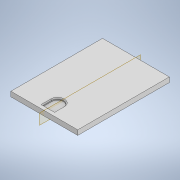
# Autodesk Inventor part: Part2
Saved by Autodesk Inventor 2022.6 (Build 266554010, 554A)
## iProperties
Created: 2025-05-13
Part Number: Part2
Material: Generic
Document SubType Name: Modeling
Designer: khinm
Density: 1 g/cm^3
Appearance: Default
Author: khinm
Autodesk Inventor part; units mm, degrees
ref_plane "XZ Plane" through (0, 0, 0) normal (0, 1, 0) x (-1, 0, 0)
ref_plane "XY Plane" through (0, 0, 0) normal (0, 0, 1) x (1, 0, 0)
sketch "Sketch1" plane through (0, 0, 0) normal (0, 0, 1) x (1, 0, 0)
  line L0 (-37.75, 2.75) -> (37.75, 2.75)
  line L1 (37.75, 2.75) -> (37.75, -2.75)
  line L2 (37.75, -2.75) -> (-37.75, -2.75)
  line L3 (-37.75, -2.75) -> (-37.75, 2.75)
  point P0 (0, 0)
  point P1 (0, 2.75)
  point P2 (-37.75, 0)
  dimension "d0" = 5.5
  dimension "d1" = 75.5
  constraints: 8 end point, 2 midpoint, 2 parallel, 1 horizontal, 1 horizontal alignment, 1 perpendicular, 1 vertical alignment
  measures "d0" distance of L0.end L1.end
  measures "d1" distance of L0.start L0.end
extrude "Extrusion1" add sketch "Sketch1" along normal mid plane 103.5
ref_plane "Work Plane1" through (0, 0, 0) normal (1, 0, 0) x (0, 1, 0)
sketch "Sketch6" plane through (0, 0, 0) normal (1, 0, 0) x (0, 1, 0)
  line L0 (-2.75, 51.75) -> (-2.75, -51.75) projected
  line L1 (-2.75, 49.5) -> (-4.75, 48.3453)
  line L2 (-4.75, 48.3453) -> (-4.75, 47.6547)
  line L3 (-4.75, 47.6547) -> (-2.75, 46.5)
  line L4 (-2.75, 46.5) -> (-2.75, 49.5)
  point P0 (0, 0)
  point P1 (-2.75, 48)
  point P2 (-4.75, 48)
  dimension "d17" = 2.25
  dimension "d18" = 3
  dimension "d19" = 2
  dimension "d20" = 60
  constraints: 8 end point, 2 midpoint, 2 parallel, 1 horizontal alignment, 1 point on line
  measures "d17" distance of L1.start L0.start
  measures "d18" distance of L3.end L1.start
  measures "d19" distance of point (-2.75, 48) point (-4.75, 48)
  measures "d20" angle of L0 L1
extrude "Extrusion4" add sketch "Sketch6" along normal mid plane 59.9
sketch "Sketch7" plane through (-37.75, 2.75, 51.75) normal (0, 1, 0) x (1, 0, 0)
  line L0 (75.5, 0) -> (0, 0) projected
  line L1 (44.3814, 15) -> (44.3814, 5)
  line L2 (44.3814, 5) -> (31.1186, 5)
  line L3 (31.1186, 5) -> (31.1186, 15)
  arc A0 (44.3814, 15) -> (31.1186, 15) centre (37.75, 15) ccw
  point P0 (37.75, 51.75)
  point P1 (37.75, 5)
  point P2 (37.75, 0)
  point P3 (37.75, 0)
  dimension "d23" = 5
  dimension "d25" = 10
  dimension "d26" = 6.6314
  constraints: 6 end point, 3 midpoint, 2 parallel, 2 point on circle, 2 vertical alignment, 1 centre point, 1 horizontal alignment
  measures "d23" distance between parallel lines of L2 L0
  measures "d25" distance of L1.end L1.start
  measures "d26" radius of A0
extrude "Extrusion5" cut sketch "Sketch7" against normal blind 2
chamfer "Chamfer2" distance 1 angle 45 4 edges at (0, 2.75, 30.1186) (6.6314, 2.75, 41.75) (-6.6314, 2.75, 41.75) (0, 2.75, 46.75)
body "Solid1"
